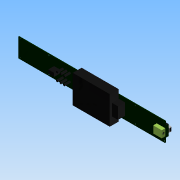
# Autodesk Inventor part: electronics
Saved by Autodesk Inventor 2015 (Build 190159000, 159)
## iProperties
Created: 2015-12-28
Part Number: electronics
Material: Générique
Document SubType Name: Modeling
Designer: Gregwar
Density: 1 g/cm^3
Appearance: Par défaut
Author: Gregwar
Autodesk Inventor part; units mm, degrees
ref_plane "YZ Plane" through (0, 0, 0) normal (1, 0, 0) x (0, 1, 0)
ref_plane "XZ Plane" through (0, 0, 0) normal (0, 1, 0) x (-1, 0, 0)
ref_plane "XY Plane" through (0, 0, 0) normal (0, 0, 1) x (1, 0, 0)
sketch "Esquisse1" plane through (0, 0, 0) normal (0, 1, 0) x (-1, 0, 0)
  line L0 (0, 0) -> (250, 0)
  line L1 (250, 0) -> (250, -32)
  line L2 (250, -32) -> (0, -32)
  line L3 (0, -32) -> (0, 0)
  circle A0 centre (2, -2) radius 1.5
  line L4 (250, -16) -> (0, -16) construction
  circle A1 centre (2, -30) radius 1.5
  circle A2 centre (51.1, -2) radius 1.5
  circle A3 centre (51.1, -30) radius 1.5
  circle A4 centre (100.2, -2) radius 1.5
  circle A5 centre (100.2, -30) radius 1.5
  circle A6 centre (149.3, -2) radius 1.5
  circle A7 centre (149.3, -30) radius 1.5
  circle A8 centre (198.4, -2) radius 1.5
  circle A9 centre (198.4, -30) radius 1.5
  circle A10 centre (247.5, -2) radius 1.5
  circle A11 centre (247.5, -30) radius 1.5
  dimension "d0" = 32
  dimension "d1" = 250
  dimension "d2" = 2
  dimension "d3" = 2
  dimension "d4" = 3
  dimension "d7" = 49.1
  constraints: 12 centre point, 10 end point, 2 horizontal, 2 midpoint, 2 parallel, 1 perpendicular, 1 symmetric about line, 21 other
  measures "d0" distance of L2.end L0.start
  measures "d1" distance of L0.start L0.end
  measures "d2" distance from line of L3 A0.centre
  measures "d3" distance from line of L0 A0.centre
  measures "d4" diameter of A0
  measures "d7" distance of A0.centre A2.centre
extrude "Extrusion1" add sketch "Esquisse1" along normal blind 1.6
sketch "Esquisse2" plane through (0, 1.6, 0) normal (0, 1, 0) x (1, 0, 0)
  circle A0 centre (-247.5, 30) radius 1.5 construction
  circle A1 centre (-247.5, 2) radius 1.5 construction
  circle A2 centre (-198.4, 30) radius 1.5 construction
  circle A3 centre (-198.4, 2) radius 1.5 construction
  circle A4 centre (-149.3, 30) radius 1.5 construction
  circle A5 centre (-149.3, 2) radius 1.5 construction
  circle A6 centre (-100.2, 30) radius 1.5 construction
  circle A7 centre (-100.2, 2) radius 1.5 construction
  circle A8 centre (-51.1, 30) radius 1.5 construction
  circle A9 centre (-51.1, 2) radius 1.5 construction
  circle A10 centre (-2, 30) radius 1.5 construction
  circle A11 centre (-2, 2) radius 1.5 construction
  line L0 (-250, 0) -> (0, 0) construction
  line L1 (0, 0) -> (0, 32) construction
  line L2 (0, 32) -> (-250, 32) construction
  line L3 (-250, 32) -> (-250, 0) construction
  line L4 (-246, 9.5) -> (-234, 9.5)
  line L5 (-234, 9.5) -> (-234, 21.5)
  line L6 (-234, 21.5) -> (-246, 21.5)
  line L7 (-246, 21.5) -> (-246, 9.5)
  dimension "d14" = 12
  dimension "d15" = 9.5
  dimension "d16" = 4
  constraints: 8 end point, 2 parallel, 2 perpendicular, 1 horizontal
  measures "d14" distance of L5.end L6.end
  measures "d15" distance between parallel lines of L0 L4
  measures "d16" distance between parallel lines of L7 L3
extrude "Extrusion2" add sketch "Esquisse2" along normal blind 7.7
sketch "Esquisse3" plane through (-246, 1.6, -21.5) normal (-1, 0, 0) x (0, 0, 1)
  circle A0 centre (4, 6) radius 1.1
  line L0 (-10.5, 0) -> (21.5, 0) projected
  line L1 (0, 0) -> (0, 7.7) projected
  line L2 (-10.5, -1.6) -> (21.5, -1.6) projected
  line L3 (5.5, -1.6) -> (5.5, 11.8569) construction
  dimension "d19" = 6
  dimension "d20" = 2.2
  dimension "d21" = 4
  constraints: 2 end point, 1 centre point, 1 midpoint, 1 vertical
  measures "d19" distance from line of L0 A0.centre
  measures "d20" diameter of A0
  measures "d21" distance from line of L1 A0.centre
extrude "Extrusion3" add sketch "Esquisse3" along normal blind 7
sketch "Esquisse4" plane through (0, 1.6, 0) normal (0, 1, 0) x (1, 0, 0)
  line L0 (-246, 9.5) -> (-246, 21.5) projected
  line L1 (-246, 21.5) -> (-234, 21.5) projected
  line L2 (-234, 21.5) -> (-234, 9.5) projected
  line L3 (-234, 9.5) -> (-246, 9.5) projected
  circle A0 centre (-247.5, 30) radius 1.5 projected
  circle A1 centre (-247.5, 2) radius 1.5 projected
  circle A2 centre (-198.4, 30) radius 1.5 projected
  circle A3 centre (-198.4, 2) radius 1.5 projected
  circle A4 centre (-149.3, 30) radius 1.5 projected
  circle A5 centre (-149.3, 2) radius 1.5 projected
  circle A6 centre (-100.2, 30) radius 1.5 projected
  circle A7 centre (-100.2, 2) radius 1.5 projected
  circle A8 centre (-51.1, 30) radius 1.5 projected
  circle A9 centre (-51.1, 2) radius 1.5 projected
  circle A10 centre (-2, 30) radius 1.5 projected
  circle A11 centre (-2, 2) radius 1.5 projected
  line L4 (-250, 0) -> (0, 0) projected
  line L5 (0, 0) -> (0, 32) projected
  line L6 (0, 32) -> (-250, 32) projected
  line L7 (-250, 32) -> (-250, 0) projected
  line L8 (0, 0) -> (0, 32) construction
  line L9 (0, 16) -> (-250, 16) construction
  line L10 (-200, 19) -> (-190, 19)
  line L11 (-190, 19) -> (-190, 13)
  line L12 (-190, 13) -> (-200, 13)
  line L13 (-200, 13) -> (-200, 19)
  line L14 (-190, 16) -> (-200, 16) construction
  line L15 (-195, 19) -> (-195, 13) construction
  dimension "d24" = 10
  dimension "d26" = 6
  dimension "d29" = 55
  constraints: 14 end point, 6 midpoint, 2 parallel, 1 collinear, 1 horizontal, 1 perpendicular
  measures "d24" distance of L10.start L10.end
  measures "d26" distance of L10.end L11.end
  measures "d29" distance between parallel lines of L15 L7
extrude "Extrusion4" add sketch "Esquisse4" along normal blind 10 contours L10 L11 L12 L13
pattern_linear "Réseau rectangulaire1" count 7 spacing 22.1667 along (1, 0, 0) of "Extrusion4"
sketch "Esquisse6" plane through (0, 0, 0) normal (0, -1, 0) x (1, 0, 0)
  line L0 (-177.8333, -13) -> (-177.8333, -19) projected
  line L1 (-190, -19) -> (-190, -13) projected
  line L2 (-188.9167, -13) -> (-178.9167, -13)
  line L3 (-178.9167, -13) -> (-178.9167, -19)
  line L4 (-178.9167, -19) -> (-188.9167, -19)
  line L5 (-188.9167, -19) -> (-188.9167, -13)
  line L6 (-188.9167, -16) -> (-178.9167, -16) construction
  line L7 (-177.8333, -19) -> (-177.8333, -13) construction
  line L8 (-177.8333, -16) -> (-190, -16) construction
  line L9 (-190, -13) -> (-190, -19) construction
  point P0 (0, 0)
  point P1 (-183.9167, -16)
  dimension "d33" = 10
  dimension "d34" = 6
  constraints: 12 end point, 6 midpoint, 2 parallel, 1 horizontal, 1 perpendicular
  measures "d33" distance of L2.start L2.end
  measures "d34" distance of L2.end L3.end
extrude "Extrusion5" add sketch "Esquisse6" along normal blind 10
sketch "Esquisse9" plane through (0, 0, 0) normal (0, -1, 0) x (1, 0, 0)
  line L0 (0, 0) -> (-250, 0) projected
  line L1 (-250, 0) -> (-250, -32) projected
  line L2 (-250, -32) -> (0, -32) projected
  line L3 (0, -32) -> (0, 0) projected
  circle A0 centre (-2, -2) radius 1.5 projected
  circle A1 centre (-2, -30) radius 1.5 projected
  circle A2 centre (-51.1, -2) radius 1.5 projected
  circle A3 centre (-51.1, -30) radius 1.5 projected
  circle A4 centre (-100.2, -30) radius 1.5 projected
  circle A5 centre (-100.2, -2) radius 1.5 projected
  circle A6 centre (-149.3, -2) radius 1.5 projected
  circle A7 centre (-149.3, -30) radius 1.5 projected
  circle A8 centre (-198.4, -2) radius 1.5 projected
  circle A9 centre (-198.4, -30) radius 1.5 projected
  circle A10 centre (-247.5, -2) radius 1.5 projected
  circle A11 centre (-247.5, -30) radius 1.5 projected
  line L4 (-178.9167, -13) -> (-178.9167, -19) projected
  line L5 (-178.9167, -19) -> (-188.9167, -19) projected
  line L6 (-188.9167, -19) -> (-188.9167, -13) projected
  line L7 (-188.9167, -13) -> (-178.9167, -13) projected
  line L8 (-178.9167, -13) -> (-178.9167, -19) construction
  line L9 (-178.9167, -16) -> (-142, -16) construction
  line L10 (-142, -1) -> (-142, -31) construction
  circle A12 centre (-173.9167, -22.5) radius 1.65
  circle A13 centre (-167.9167, -22.5) radius 1.65
  circle A14 centre (-161.9167, -22.5) radius 1.65
  circle A15 centre (-173.9167, -9.5) radius 1.65
  circle A16 centre (-167.9167, -9.5) radius 1.65
  circle A17 centre (-161.9167, -9.5) radius 1.65
  dimension "d51" = 6
  dimension "d56" = 3.3
  dimension "d57" = 13
  dimension "d58" = 5
  constraints: 6 centre point, 3 symmetric about line, 2 end point, 2 midpoint, 1 horizontal, 7 other
  measures "d51" distance of A12.centre A13.centre
  measures "d56" diameter of A15
  measures "d57" distance of A12.centre A15.centre
  measures "d58" distance from line of L4 A15.centre
extrude "Extrusion8" add sketch "Esquisse9" along normal blind 10 contours A12 | A13 | A14 | A15 | A16 | A17
sketch "Esquisse11" plane through (0, 1.6, 0) normal (0, 1, 0) x (1, 0, 0)
  line L0 (-57, 19) -> (-57, 13) projected
  line L1 (-57, 13) -> (-67, 13) projected
  line L2 (-67, 13) -> (-67, 19) projected
  line L3 (-67, 19) -> (-57, 19) projected
  line L4 (-79.1667, 19) -> (-79.1667, 13) projected
  line L5 (-79.1667, 13) -> (-89.1667, 13) projected
  line L6 (-89.1667, 13) -> (-89.1667, 19) projected
  line L7 (-89.1667, 19) -> (-79.1667, 19) projected
  line L8 (-101.3333, 19) -> (-101.3333, 13) projected
  line L9 (-101.3333, 13) -> (-111.3333, 13) projected
  line L10 (-111.3333, 13) -> (-111.3333, 19) projected
  line L11 (-111.3333, 19) -> (-101.3333, 19) projected
  line L12 (-123.5, 19) -> (-123.5, 13) projected
  line L13 (-123.5, 13) -> (-133.5, 13) projected
  line L14 (-133.5, 13) -> (-133.5, 19) projected
  line L15 (-133.5, 19) -> (-123.5, 19) projected
  line L16 (-145.6667, 19) -> (-145.6667, 13) projected
  line L17 (-145.6667, 13) -> (-155.6667, 13) projected
  line L18 (-155.6667, 13) -> (-155.6667, 19) projected
  line L19 (-155.6667, 19) -> (-145.6667, 19) projected
  line L20 (-167.8333, 19) -> (-167.8333, 13) projected
  line L21 (-167.8333, 13) -> (-177.8333, 13) projected
  line L22 (-177.8333, 13) -> (-177.8333, 19) projected
  line L23 (-177.8333, 19) -> (-167.8333, 19) projected
  line L24 (-190, 19) -> (-190, 13) projected
  line L25 (-190, 13) -> (-200, 13) projected
  line L26 (-200, 13) -> (-200, 19) projected
  line L27 (-200, 19) -> (-190, 19) projected
  line L28 (-246, 9.5) -> (-246, 21.5) projected
  line L29 (-246, 21.5) -> (-234, 21.5) projected
  line L30 (-234, 21.5) -> (-234, 9.5) projected
  line L31 (-234, 9.5) -> (-246, 9.5) projected
  circle A0 centre (-247.5, 30) radius 1.5 projected
  circle A1 centre (-247.5, 2) radius 1.5 projected
  circle A2 centre (-198.4, 30) radius 1.5 projected
  circle A3 centre (-198.4, 2) radius 1.5 projected
  circle A4 centre (-149.3, 30) radius 1.5 projected
  circle A5 centre (-149.3, 2) radius 1.5 projected
  circle A6 centre (-100.2, 30) radius 1.5 projected
  circle A7 centre (-100.2, 2) radius 1.5 projected
  circle A8 centre (-51.1, 30) radius 1.5 projected
  circle A9 centre (-51.1, 2) radius 1.5 projected
  circle A10 centre (-2, 30) radius 1.5 projected
  circle A11 centre (-2, 2) radius 1.5 projected
  line L32 (-250, 0) -> (0, 0) projected
  line L33 (0, 0) -> (0, 32) projected
  line L34 (0, 32) -> (-250, 32) projected
  line L35 (-250, 32) -> (-250, 0) projected
  line L36 (-52, 25) -> (0, 25)
  line L37 (0, 25) -> (0, 7)
  line L38 (0, 7) -> (-52, 7)
  line L39 (-52, 7) -> (-52, 25)
  line L40 (-52, 16) -> (0, 16) construction
  line L41 (0, 0) -> (0, 32) construction
  line L42 (0, 16) -> (-57, 16) construction
  line L43 (-57, 19) -> (-57, 13) construction
  dimension "d61" = 18
  dimension "d62" = 52
  constraints: 12 end point, 4 midpoint, 2 collinear, 2 parallel, 1 horizontal, 1 perpendicular
  measures "d61" distance between parallel lines of L38 L36
  measures "d62" distance of L36.start L36.end
extrude "Extrusion9" add sketch "Esquisse11" along normal blind 4.5 contours L38 L39 L36 L33
sketch "Esquisse12" plane through (0, 6.1, 0) normal (0, 1, 0) x (1, 0, 0)
  line L0 (0, 25) -> (-52, 25) projected
  line L1 (-52, 25) -> (-52, 7) projected
  line L2 (-52, 7) -> (0, 7) projected
  line L3 (0, 7) -> (0, 25) projected
  line L4 (0, 32) -> (0, 0) construction
  line L5 (0, 16) -> (-52, 16) construction
  line L6 (-52, 25) -> (-52, 7) construction
  line L7 (-7.5, 12.25) -> (0, 12.25)
  line L8 (0, 12.25) -> (0, 19.75)
  line L9 (0, 19.75) -> (-7.5, 19.75)
  line L10 (-7.5, 19.75) -> (-7.5, 12.25)
  line L11 (0, 19.75) -> (1, 19.75)
  line L12 (1, 19.75) -> (1, 12.25)
  line L13 (1, 12.25) -> (0, 12.25)
  line L14 (0, 12.25) -> (0, 19.75)
  point P0 (0, 16)
  dimension "d65" = 7.5
  dimension "d66" = 7.5
  dimension "d69" = 1
  constraints: 18 end point, 4 midpoint, 4 parallel, 2 horizontal, 2 perpendicular
  measures "d65" distance between parallel lines of L7 L9
  measures "d66" distance of L8.end L9.end
  measures "d69" distance of L8.end L11.end
extrude "Extrusion10" add sketch "Esquisse12" along normal blind 4 contours L11 L12 L13 L3 | L3 L7 L10 L9
sketch "Esquisse13" plane through (1, 6.1, -12.25) normal (1, 0, 0) x (0, 0, -1)
  line L0 (0, 0) -> (7.5, 0) projected
  line L1 (7.5, 0) -> (7.5, 4) projected
  line L2 (0, 4) -> (7.5, 4) projected
  line L3 (0, 0) -> (0, 4) projected
  line L4 (0.5, 3.5) -> (7, 3.5)
  line L5 (7, 3.5) -> (6.25, 0.5)
  line L6 (6.25, 0.5) -> (1.25, 0.5)
  line L7 (1.25, 0.5) -> (0.5, 3.5)
  line L8 (3.75, 3.5) -> (3.75, 0.5) construction
  line L9 (7.5, 4) -> (0, 4) construction
  line L10 (3.75, 4) -> (3.75, 0) construction
  line L11 (12.75, 0) -> (-5.25, 0) construction
  point P0 (-12.25, -6.1)
  dimension "d71" = 0.5
  dimension "d72" = 0.5
  dimension "d73" = 0.5
  dimension "d74" = 5
  constraints: 12 end point, 4 midpoint, 2 perpendicular, 1 collinear, 1 horizontal
  measures "d71" distance between parallel lines of L4 L2
  measures "d72" distance between parallel lines of L0 L6
  measures "d73" distance from line of L1 L4.end
  measures "d74" distance of L5.end L6.end
extrude "Extrusion11" cut sketch "Esquisse13" against normal blind 3 contours L4 L5 L6 L7
sketch "Esquisse14" plane through (0, 0, 0) normal (0, -1, 0) x (1, 0, 0)
  line L0 (0, -10) -> (-14, -10)
  line L1 (-14, -10) -> (-14, -22)
  line L2 (-14, -22) -> (0, -22)
  line L3 (0, -22) -> (0, -10)
  line L4 (0, -12.25) -> (0, -19.75) construction
  line L5 (0, -16) -> (-15.2374, -16) construction
  line L6 (0, -16) -> (-14, -16) construction
  line L7 (0, -32) -> (0, 0) construction
  line L8 (0.5, -22) -> (0, -22)
  line L9 (0, -22) -> (0, -10)
  line L10 (0, -10) -> (0.5, -10)
  line L11 (0.5, -10) -> (0.5, -22)
  dimension "d77" = 12
  dimension "d78" = 14
  dimension "d85" = 0.5
  constraints: 20 end point, 4 midpoint, 4 parallel, 3 horizontal, 2 perpendicular, 1 collinear
  measures "d77" distance between parallel lines of L2 L0
  measures "d78" distance of L1.end L2.end
  measures "d85" distance of L8.start L2.end
extrude "Extrusion12" add sketch "Esquisse14" along normal blind 6
sketch "Esquisse15" plane through (0, 0, -32) normal (1, 0, 0) x (0, 0, -1)
  line L0 (0, 0) -> (-10, 0) projected
  line L1 (0, 0) -> (0, 1.6) projected
  line L2 (-7, 1.6) -> (0, 1.6) projected
  line L3 (-7, 1.6) -> (-7, 6.1) projected
  line L4 (-12.25, 6.1) -> (-7, 6.1) projected
  line L5 (-19.75, 6.1) -> (-12.25, 6.1) projected
  line L6 (-25, 6.1) -> (-19.75, 6.1) projected
  line L7 (-25, 1.6) -> (-25, 6.1) projected
  line L8 (-32, 1.6) -> (-25, 1.6) projected
  line L9 (-32, 0) -> (-32, 1.6) projected
  line L10 (-22, -6) -> (-10, -6) construction
  line L11 (-16, -6) -> (-16, -0.2) construction
  circle A0 centre (-16, -3) radius 1.7
  line L12 (-10, 0) -> (-22, 0) construction
  line L13 (-22, 0) -> (-32, 0) projected
  line L14 (-10, 0) -> (-22, 0) projected
  dimension "d81" = 3
  dimension "d82" = 3.4
  constraints: 2 end point, 1 centre point, 1 midpoint, 1 point on line, 1 vertical
  measures "d81" distance from line of L12 A0.centre
  measures "d82" diameter of A0
extrude "Extrusion13" cut sketch "Esquisse15" along normal mid plane 40 contours A0
sketch "Esquisse16" plane through (0, 0, 0) normal (0, -1, 0) x (1, 0, 0)
  line L0 (-142, 8) -> (-79, 8)
  line L1 (-79, 8) -> (-79, -40)
  line L2 (-79, -40) -> (-142, -40)
  line L3 (-142, -40) -> (-142, 8)
  line L4 (-79, -16) -> (-142, -16) construction
  line L5 (-250, 0) -> (-250, -32) construction
  line L6 (-250, -16) -> (0, -16) construction
  line L7 (0, -32) -> (0, -22) construction
  line L8 (-14, -10) -> (-14, -22) construction
  point P0 (0, 0)
  dimension "d86" = 63
  dimension "d87" = 48
  dimension "d91" = 108
  constraints: 12 end point, 3 midpoint, 2 parallel, 2 perpendicular, 1 collinear, 1 horizontal, 1 point on line
  measures "d86" distance of L0.start L0.end
  measures "d87" distance of L0.end L1.end
  measures "d91" distance between parallel lines of L3 L5
extrude "Extrusion14" add sketch "Esquisse16" along normal blind 15
sketch "Esquisse17" plane through (0, 0, 0) normal (0, -1, 0) x (1, 0, 0)
  line L0 (-78, -26) -> (-68, -26)
  line L1 (-68, -26) -> (-68, -6)
  line L2 (-68, -6) -> (-78, -6)
  line L3 (-78, -6) -> (-78, -26)
  line L4 (-14, -22) -> (-14, -10) construction
  line L5 (-14, -16) -> (-79, -16) construction
  line L6 (-79, 0) -> (-79, -32) construction
  line L7 (-78, -16) -> (-68, -16) construction
  line L8 (0, -10) -> (0, 0) construction
  dimension "d92" = 68
  dimension "d93" = 10
  dimension "d94" = 20
  constraints: 12 end point, 4 midpoint, 2 parallel, 1 collinear, 1 horizontal, 1 perpendicular
  measures "d92" distance between parallel lines of L8 L1
  measures "d93" distance of L0.start L0.end
  measures "d94" distance of L2.end L0.start
extrude "Extrusion15" add sketch "Esquisse17" along normal blind 12
equation "\"d72\" = d71"
equation "\"d73\" = d71"
